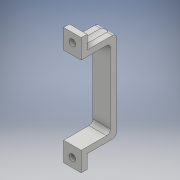
# Autodesk Inventor part: esc-bracket
Saved by Autodesk Inventor 2018 (Build 220112000, 112)
## iProperties
Created: 2017-10-22
Part Number: esc-bracket
Material: Generic
Document SubType Name: Modeling
Designer: leo2a
Density: 1 g/cm^3
Appearance: Default
Author: leo2a
Autodesk Inventor part; units mm, degrees
ref_plane "YZ Plane" through (0, 0, 0) normal (1, 0, 0) x (0, 1, 0)
ref_plane "XZ Plane" through (0, 0, 0) normal (0, 1, 0) x (-1, 0, 0)
ref_plane "XY Plane" through (0, 0, 0) normal (0, 0, 1) x (1, 0, 0)
sketch "Sketch1" plane through (0, 0, 0) normal (1, 0, 0) x (0, 1, 0)
  line L0 (0, 0) -> (0, 20)
  line L1 (0, 20) -> (-15, 20)
  line L2 (0, 0) -> (3, 0)
  line L3 (3, 0) -> (3, 23)
  line L4 (3, 23) -> (-12, 23)
  line L5 (-12, 23) -> (-12, 28)
  line L6 (-12, 28) -> (-15, 28)
  line L7 (-15, 28) -> (-15, 20)
  line L8 (3.6548, 0) -> (-1.246, 0)
  line L9 (0, 0) -> (0, -20)
  line L10 (0, -20) -> (-15, -20)
  line L11 (3, 0) -> (3, -23)
  line L12 (3, -23) -> (-12, -23)
  line L13 (-12, -23) -> (-12, -28)
  line L14 (-15, -28) -> (-15, -20)
  line L15 (-12, -28) -> (-15, -28)
  line L16 (-12, 28) -> (-12, 30)
  line L17 (-12, 30) -> (-15, 30)
  line L18 (-15, 30) -> (-15, 28)
  line L19 (-15, -28) -> (-15, -30)
  line L20 (-15, -30) -> (-12, -30)
  line L21 (-12, -30) -> (-12, -28)
  dimension "d0" = 20
  dimension "d1" = 15
  dimension "d2" = 3
  dimension "d3" = 23
  dimension "d4" = 15
  dimension "d5" = 5
  dimension "d22" = 2
  dimension "d23" = 2
  constraints: 44 end point, 10 perpendicular, 6 symmetric about line, 3 vertical, 2 horizontal, 2 point on line
  measures "d0" distance of L0.start L0.end
  measures "d1" distance of L0.end L1.end
  measures "d2" distance of L0.start L2.end
  measures "d3" distance of L2.end L3.end
  measures "d4" distance of L3.end L4.end
  measures "d5" distance of L4.end L5.end
  measures "d22" distance of L5.end L16.end
  measures "d23" distance of L14.start L19.end
extrude "Extrusion1" add sketch "Sketch1" along normal blind 7 and the other way blind 2
sketch "Sketch2" plane through (0, -12, 28) normal (0, 1, 0) x (1, 0, 0)
  line L0 (0, 0) -> (-2, 2.1)
  line L1 (-2, -2) -> (-2, 5) projected
  line L2 (-2, 58) -> (-2, 48) projected
  line L3 (0, 56) -> (-2, 54.5)
  point P0 (0, 28)
  point P1 (2.5, 2.5)
  point P2 (2.5, 53.5)
  dimension "d8" = 2.9
  dimension "d9" = 2.5
  constraints: 4 end point, 4 other
  measures "d8" distance of L0.start L0.end
  measures "d9" distance of L3.start L3.end
hole "Hole1" at (2.5, -12, 25.5) at (2.5, -12, -25.5) direction (0, -1, 0) diameter 3.4 end through all clearance for "Countersunk Flat Head Screw ISO 2009/7046" size "M3" standard "ISO"
sketch "Sketch3" plane through (0, -12, 28) normal (0, 1, 0) x (1, 0, 0)
  circle A0 centre (2.5, 2.5) radius 1.7 projected
  circle A1 centre (2.5, 2.5) radius 3
  circle A2 centre (2.5, 53.5) radius 1.7 projected
  circle A3 centre (2.5, 53.5) radius 3
  point P0 (0, 28)
  dimension "d17" = 6
  dimension "d18" = 6
  constraints: 2 centre point, 2 coincident
  measures "d17" diameter of A1
  measures "d18" diameter of A3
fillet "Fillet1" radius 2 4 edges at (2.5, 3, 23) (2.5, 0, 20) (2.5, 0, -20) (2.5, 3, -23)
extrude "Extrusion2" cut sketch "Sketch3" along normal blind 20
body "Solid1"
